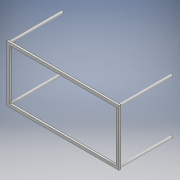
# Autodesk Inventor part: LedSystem
Saved by Autodesk Inventor 2017 (Build 210142000, 142)
## iProperties
Created: 2016-11-27
Part Number: LedSystem
Material: Generic
Document SubType Name: Modeling
Designer: umr
Density: 1 g/cm^3
Appearance: Default
Author: umr
Autodesk Inventor part; units mm, degrees
ref_plane "YZ Plane" through (0, 0, 0) normal (1, 0, 0) x (0, 1, 0)
ref_plane "XZ Plane" through (0, 0, 0) normal (0, 1, 0) x (-1, 0, 0)
ref_plane "XY Plane" through (0, 0, 0) normal (0, 0, 1) x (1, 0, 0)
sketch "Sketch1" plane through (0, 0, 0) normal (0, 1, 0) x (-1, 0, 0)
  line L0 (0, 0) -> (3000, 0)
  line L1 (3000, 0) -> (3000, -1500)
  line L2 (3000, -1500) -> (0, -1500)
  line L3 (0, -1500) -> (0, 0)
  line L4 (75, -75) -> (2925, -75)
  line L5 (2925, -75) -> (2925, -1425)
  line L6 (2925, -1425) -> (75, -1425)
  line L7 (75, -1425) -> (75, -75)
  dimension "d0" = 3000
  dimension "d1" = 1500
  dimension "d2" = 75
  dimension "d3" = 1350
  dimension "d4" = 75
  dimension "d5" = 2850
  constraints: 16 end point, 4 parallel, 2 horizontal, 2 perpendicular
  measures "d0" distance of L1.end L2.end
  measures "d1" distance of L0.end L1.end
  measures "d2" distance between parallel lines of L0 L4
  measures "d3" distance of L4.end L5.end
  measures "d4" distance between parallel lines of L1 L5
  measures "d5" distance of L5.end L6.end
extrude "Extrusion1" add sketch "Sketch1" along normal blind 50
sketch "Sketch2" plane through (0, 50, 0) normal (0, 1, 0) x (1, 0, 0)
  circle A0 centre (-2962.5, 37.5) radius 30
  line L0 (-3000, 0) -> (0, 0) projected
  line L1 (-75, 75) -> (-2925, 75) projected
  line L2 (-3000, 1500) -> (-3000, 0) projected
  line L3 (-2925, 75) -> (-2925, 1425) projected
  line L4 (-1500, 750) -> (-3750.0767, 750)
  line L5 (-1500, 750) -> (-1500, 2776.2383)
  circle A1 centre (-2962.5, 1462.5) radius 30
  circle A2 centre (-37.5, 37.5) radius 30
  circle A3 centre (-37.5, 1462.5) radius 30
  dimension "d8" = 75
  dimension "d9" = 60
  dimension "d10" = 37.5
  dimension "d11" = 75
  dimension "d12" = 37.5
  constraints: 4 centre point, 4 end point, 3 symmetric about line, 1 horizontal, 1 vertical, 3 other
  measures "d8" distance between parallel lines of L0 L1
  measures "d9" diameter of A0
  measures "d10" distance from line of L0 A0.centre
  measures "d11" distance between parallel lines of L2 L3
  measures "d12" distance from line of L2 A0.centre
extrude "Extrusion2" add sketch "Sketch2" along normal blind 1400
equation "\"d2\" = 0.05 * d1"
equation "\"d3\" = d1 - 2 * d2"
equation "\"d4\" = 0.025 * d0"
equation "\"d5\" = d0 - 2 * d4"
equation "\"d9\" = 0.8 * d8"
equation "\"d10\" = 0.5 * d8 + 0 * d9"
equation "\"d12\" = 0.5 * d11 + 0 * d9"
body "Solid1"
